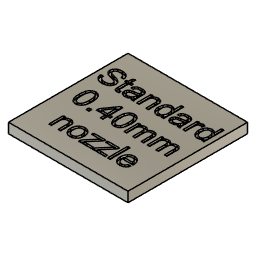
Labelled Swatch (Autodesk Fusion 360 design; units mm, degrees)
Autodesk Fusion 360 part; units mm, degrees
sketch "Create swatch" plane through (0, 0, 0) normal (0, 0, 1) x (1, 0, 0)
  line L0 (0, 0) -> (60, 0)
  line L1 (60, 0) -> (60, 60)
  line L2 (60, 60) -> (0, 60)
  line L3 (0, 60) -> (0, 0)
  dimension "d7" = 60
  dimension "d8" = 60
  constraint horizontal L0
  constraint vertical L1
  constraint horizontal L2
  constraint vertical L3
  constraint coincident L0.start L3.end
  measures "d7" distance of L0.start L0.end
  measures "d8" distance of L0.start L2.end
extrude "Extrude1" add sketch "Create swatch" along normal blind 5
sketch "Add label" plane through (0, 0, 5) normal (0, 0, 1) x (-1, 0, 0)
  line L0 (0, -60) -> (0, 0)
  line L1 (0, 0) -> (-60, 0)
  line L2 (-60, 0) -> (-60, -60)
  line L3 (-60, -60) -> (0, -60)
  line L4 (0, 0) -> (-60, 0) construction
  line L5 (-60, 0) -> (-60, -60) construction
  line L6 (-60, -60) -> (0, -60) construction
  line L7 (0, -60) -> (0, 0) construction
  dimension "d46" = 10
  text T0 "Standard 0.40mm nozzle" font "Arial" height 10 align centre middle in box 60 x 60 at (0, 0) x (-1, 0) y (0, -1) spacing 1
  constraint coincident L1.end
  constraint coincident L0.start
extrude "Extrude11" cut sketch "Add label" against normal blind 1 text T0
equation "SwatchWidth = 60 mm" comment "Width of swatch block"
equation "SwatchDepth = 60 mm" comment "Depth of swatch block"
equation "SwatchHeight = 5 mm" comment "Thickness of main test block"
equation "d7 = SwatchWidth"
equation "d8 = SwatchDepth"
equation "d9 = SwatchHeight"
equation "EngraveDepth = 1 mm"
equation "d50 = -EngraveDepth"
named bodies: "Swatch"
